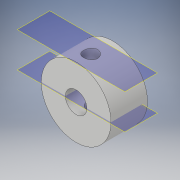
# Autodesk Inventor part: brImp_fan
Saved by Autodesk Inventor 2018 (Build 220112000, 112)
## iProperties
Created: 2018-02-04
Part Number: brImp_fan
Material: Generic
Document SubType Name: Modeling
Designer: Benedikt
Density: 1 g/cm^3
Appearance: Default
Author: Benedikt
## iProperties of the stored document brImp_fan_3DPrint.ipt
Created: 2018-02-04
Part Number: brImp_fan_3DPrint
Material: Generic
Document SubType Name: Modeling
Designer: Benedikt
Density: 1 g/cm^3
Appearance: Default
Author: Benedikt
Autodesk Inventor part; units mm, degrees
ref_plane "YZ Plane" through (0, 0, 0) normal (1, 0, 0) x (0, 1, 0)
ref_plane "XZ Plane" through (0, 0, 0) normal (0, 1, 0) x (-1, 0, 0)
ref_plane "XY Plane" through (0, 0, 0) normal (0, 0, 1) x (1, 0, 0)
sketch "Sketch1" plane through (0, 0, 0) normal (0, 1, 0) x (-1, 0, 0)
  circle A0 centre (0, 0) radius 15.3
  circle A1 centre (0, 0) radius 4.7
  dimension "d0" = 30.6
  dimension "d1" = 9.4
  constraints: 2 centre point, 2 coincident
  measures "d0" diameter of A0
  measures "d1" diameter of A1
extrude "Extrusion1" add sketch "Sketch1" along normal blind 13
sketch "Sketch2" plane through (0, 13, 0) normal (0, 1, 0) x (1, 0, 0)
  line L0 (19.8933, 0) -> (-23.0575, 0) construction
  point P0 (0, 0)
  constraints: 2 end point, 1 horizontal
ref_plane "Work Plane1" through (19.8933, 13, 0) normal (0, 0, -1) x (-1, 0, 0)
sketch "Sketch3" plane through (19.8933, 13, 0) normal (0, 0, -1) x (-1, 0, 0)
  circle A0 centre (19.8933, -6.75) radius 1.95
  line L0 (35.1933, 0) -> (4.5933, 0) projected
  line L1 (15.1933, 0) -> (24.5933, 0) projected
  point P0 (19.8933, -13)
  dimension "d5" = 3.9
  dimension "d18" = 6.75
  constraints: 1 centre point, 1 coincident
  measures "d5" diameter of A0
  measures "d18" distance from line of L1 A0.centre
extrude "Extrusion2" cut sketch "Sketch3" along normal through all both and the other way through all
ref_plane "Work Plane2" through (0, 0, 15.3) normal (0, 0, -1) x (-1, 0, 0)
sketch "Sketch4" plane through (0, 0, 15.3) normal (0, 0, -1) x (-1, 0, 0)
  point P0 (0, 0)
  point P1 (1.95, 6.25)
  point P2 (0, 6.35)
  constraints: 1 other
hole "Hole1" at (0, 6.35, 15.3) direction (0, 0, -1) diameter 6.2 depth 6.5 tip angle 118
mirror "Mirror1" about plane through (19.8933, 13, 0) normal (0, 0, -1) of "Hole1"
sketch "Sketch5" plane through (0, 13, 0) normal (0, 1, 0) x (1, 0, 0)
  circle A0 centre (0, 0) radius 15.3 projected
extrude "Extrusion3" add sketch "Sketch5" along normal blind 3
body "Solid1"
